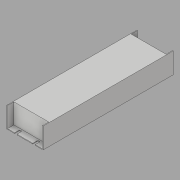
# Autodesk Inventor part: UHP-1500-230
Saved by Autodesk Inventor 2017 (Build 210142000, 142)
## iProperties
Created: 2022-09-19
Part Number: UHP-1500-230
Material: Generic
Document SubType Name: Modeling
Designer: JTS
Density: 1 g/cm^3
Appearance: Default
Author: JTS
Autodesk Inventor part; units mm, degrees
ref_plane "YZ Plane" through (0, 0, 0) normal (1, 0, 0) x (0, 1, 0)
ref_plane "XZ Plane" through (0, 0, 0) normal (0, 1, 0) x (-1, 0, 0)
sketch "Sketch1" plane through (0, 0, 0) normal (0, 0, 1) x (1, 0, 0)
  line L0 (-34, -19.4) -> (34, -19.4)
  line L1 (34, -19.4) -> (34, 19.4)
  line L2 (34, 19.4) -> (-34, 19.4)
  line L3 (-34, 19.4) -> (-34, -19.4)
  line L4 (-34, -19.4) -> (34, 19.4) construction
  line L5 (34, -19.4) -> (-34, 19.4) construction
  point P0 (0, 0)
  dimension "d0" = 68
  dimension "d1" = 38.8
  constraints: 12 end point, 2 horizontal, 2 midpoint, 2 vertical
  measures "d0" distance of L0.start L0.end
  measures "d1" distance of L2.end L0.start
extrude "Extrusion1" add sketch "Sketch1" along normal blind 244.2
sketch "Sketch2" plane through (-34, 19.4, 0) normal (0, 1, 0) x (1, 0, 0)
  line L0 (68, -244.2) -> (0, -244.2) projected
  line L1 (68, 0) -> (0, 0) projected
  arc A0 (19.15, -236.7) -> (14.65, -236.7) centre (16.9, -236.7) ccw
  arc A1 (53.35, -236.7) -> (48.85, -236.7) centre (51.1, -236.7) ccw
  arc A2 (48.85, -7.5) -> (53.35, -7.5) centre (51.1, -7.5) ccw
  arc A3 (14.65, -7.5) -> (19.15, -7.5) centre (16.9, -7.5) ccw
  line L2 (16.9, -236.7) -> (16.9, -7.5) construction
  line L3 (16.9, -7.5) -> (51.1, -7.5) construction
  line L4 (51.1, -7.5) -> (51.1, -236.7) construction
  line L5 (16.9, -236.7) -> (16.9, -244.2) construction
  line L6 (16.9, -7.5) -> (16.9, 0) construction
  line L7 (16.9, -7.5) -> (0, 0) construction
  line L8 (51.1, -7.5) -> (68, 0) construction
  line L9 (48.85, -236.7) -> (48.85, -244.2)
  line L10 (53.35, -236.7) -> (53.35, -244.2)
  line L11 (14.65, -236.7) -> (14.65, -244.2)
  line L12 (19.15, -236.7) -> (19.15, -244.2)
  line L13 (19.15, -7.5) -> (19.15, 0)
  line L14 (14.65, -7.5) -> (14.65, 0)
  line L15 (53.35, -7.5) -> (53.35, 0)
  line L16 (48.85, -7.5) -> (48.85, 0)
  point P0 (34, 0)
  dimension "d4" = 2.25
  dimension "d5" = 229.2
  dimension "d6" = 34.2
  constraints: 30 end point, 12 vertical, 10 point on line, 8 point on circle, 8 tangent, 4 centre point, 3 equal length, 3 equal radius, 1 coincident, 1 horizontal
  measures "d4" radius of A3
  measures "d5" distance of L2.start L2.end
  measures "d6" distance of L2.end L3.end
extrude "Extrusion2" cut sketch "Sketch2" against normal up to surface (38.8 mm away)
ref_plane "Work Plane1" through (34, -18.13, 0) normal (0, -1, 0) x (1, 0, 0)
sketch "Sketch3" plane through (-34, 19.4, 244.2) normal (0, 1, 0) x (1, 0, 0)
  line L0 (0, 244.2) -> (0, 0) projected
  line L1 (68, 244.2) -> (68, 0) projected
  line L2 (66.73, 0) -> (66.73, 12)
  line L3 (66.73, 12) -> (1.27, 12)
  line L4 (1.27, 12) -> (1.27, 0)
  line L5 (1.27, 0) -> (66.73, 0)
  line L6 (1.27, 0) -> (0, 0) construction
  line L7 (68, 0) -> (66.73, 0) construction
  line L8 (1.27, 232.2) -> (66.73, 232.2)
  line L9 (66.73, 232.2) -> (66.73, 244.2)
  line L10 (66.73, 244.2) -> (1.27, 244.2)
  line L11 (1.27, 244.2) -> (1.27, 232.2)
  line L12 (1.27, 244.2) -> (0, 244.2) construction
  point P0 (34, 244.2)
  dimension "d9" = 1.27
  dimension "d14" = 220.2
  constraints: 22 end point, 6 horizontal, 4 collinear, 2 vertical
  measures "d9" distance of L4.end L0.end
  measures "d14" distance between parallel lines of L3 L8
extrude "Extrusion3" cut sketch "Sketch3" against normal up to surface (37.53 mm away)
body "Solid1"
